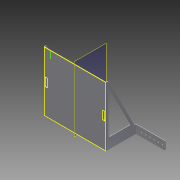
# Autodesk Inventor part: battery mount
Saved by Autodesk Inventor 2014 SP1 (Build 180222100, 222)
## iProperties
Created: 2014-01-05
Part Number: battery mount
Material: Aluminum 6061
Document SubType Name: Sheet Metal
Designer: Arpan
Density: 2.71 g/cm^3
Flat Pattern Width: 54.6969 cm
Flat Pattern Length: 18.034 cm
Flat Pattern Area: 986.403 cm^2
Sheet Metal Rule: Default
Sheet Metal Width: 21.534 in
Sheet Metal Length: 7.100 in
Sheet Metal Area: 152.893 in^2
Appearance: Aluminum - Flat
Mass: 205.427 g
Surface Area: 991.477 cm^2
Volume: 75.8033 cm^3
Author: Arpan
Autodesk Inventor part; units mm, degrees
ref_plane "YZ Plane" through (0, 0, 0) normal (1, 0, 0) x (0, 1, 0)
ref_plane "XZ Plane" through (0, 0, 0) normal (0, 1, 0) x (-1, 0, 0)
ref_plane "XY Plane" through (0, 0, 0) normal (0, 0, 1) x (1, 0, 0)
sketch "Sketch1" plane through (0, 0, 0) normal (0, 0, 1) x (1, 0, 0)
  line L0 (0, 0) -> (-186.69, 0)
  line L1 (-186.69, 0) -> (-186.69, 180.34)
  line L2 (-186.69, 180.34) -> (0, 180.34)
  line L3 (0, 180.34) -> (0, 0)
  line L4 (-186.69, 90.17) -> (-183.515, 90.17)
  line L5 (-183.515, 90.17) -> (-183.515, 102.87)
  line L6 (-183.515, 102.87) -> (-177.165, 102.87)
  line L7 (-177.165, 102.87) -> (-177.165, 77.47)
  line L8 (-177.165, 77.47) -> (-183.515, 77.47)
  line L9 (-183.515, 77.47) -> (-183.515, 90.17)
  line L10 (0, 90.17) -> (-3.175, 90.17)
  line L11 (-3.175, 90.17) -> (-3.175, 102.87)
  line L12 (-3.175, 102.87) -> (-9.525, 102.87)
  line L13 (-9.525, 102.87) -> (-9.525, 77.47)
  line L14 (-9.525, 77.47) -> (-3.175, 77.47)
  line L15 (-3.175, 77.47) -> (-3.175, 90.17)
  dimension "d0" = 180.34
  dimension "d1" = 186.69
  dimension "d2" = 3.175
  dimension "d3" = 12.7
  dimension "d4" = 6.35
  dimension "d5" = 25.4
  dimension "d6" = 3.175
  dimension "d7" = 6.35
  dimension "d8" = 25.4
  measures "d0" distance of L2.end L0.start
  measures "d1" distance of L0.start L0.end
  measures "d2" distance of L4.start L4.end
  measures "d3" distance of L4.end L5.end
  measures "d4" distance of L5.end L6.end
  measures "d5" distance of L6.end L7.end
  measures "d6" distance of L10.start L10.end
  measures "d7" distance of L11.end L12.end
  measures "d8" distance of L12.end L13.end
extrude "Plate1" add sketch "Sketch1" along normal blind 1.5875
sketch "Sketch2" plane through (0.127, 0, -0.127) normal (1, 0, 0) x (0, 1, 0)
  line L0 (180.34, 0) -> (0, 0)
  line L1 (0, 0) -> (0, -88.773)
  line L2 (0, -88.773) -> (180.34, -88.773)
  line L3 (180.34, -88.773) -> (180.34, 0)
  constraints: 6 end point, 1 horizontal, 1 perpendicular, 1 vertical
edge flange "Flange1" height 88.9 angle 90 thickness 1.5875 bend radius 0.127 thickness toward (1, 0, 0) relief straight relief width 1.5875 relief depth 0.7937 corner gap 1.5875 corner form 0 edges at (0, 45.085, 0) (0, 135.255, 0) wall of the first edge with corners at (0.127, 180.34, -0.127) (0.127, 0, -0.127) (0.127, 0, -88.9) (0.127, 180.34, -88.9)
bend "Bend1"
corner "Corner1"
sketch "Sketch3" plane through (-186.817, 180.34, -0.127) normal (-1, 0, 0) x (0, -1, 0)
  line L0 (180.34, 0) -> (0, 0)
  line L1 (0, 0) -> (0, -88.773)
  line L2 (0, -88.773) -> (180.34, -88.773)
  line L3 (180.34, -88.773) -> (180.34, 0)
  constraints: 6 end point, 1 horizontal, 1 perpendicular, 1 vertical
edge flange "Flange2" height 88.9 angle 90 thickness 1.5875 bend radius 0.127 thickness toward (-1, 0, 0) relief straight relief width 1.5875 relief depth 0.7937 edges at (-186.69, 90.17, 0) wall of the first edge with corners at (-186.817, 0, -0.127) (-186.817, 180.34, -0.127) (-186.817, 180.34, -88.9) (-186.817, 0, -88.9)
bend "Bend2"
corner "Corner2"
sketch "Sketch4" plane through (1.8415, 180.34, -89.027) normal (0, 0, -1) x (-1, 0, 0)
  line L0 (0, -180.34) -> (0, 0)
  line L1 (0, 0) -> (-88.773, 0)
  line L2 (-88.773, 0) -> (-88.773, -180.34)
  line L3 (-88.773, -180.34) -> (0, -180.34)
  constraints: 6 end point, 1 horizontal, 1 perpendicular, 1 vertical
edge flange "Flange3" height 88.9 angle 90 thickness 1.5875 bend radius 0.127 thickness toward (0, 0, -1) relief straight relief width 1.5875 relief depth 0.7937 corner gap 1.5875 corner form 0 edges at (1.7145, 90.17, -88.9) (-188.4045, 90.17, -88.9) wall of the first edge with corners at (1.8415, 0, -89.027) (1.8415, 180.34, -89.027) (90.6145, 180.34, -89.027) (90.6145, 0, -89.027)
bend "Bend3"
corner "Corner3"
sketch "Sketch5" plane through (-277.3045, 0, -90.6145) normal (0, 0, -1) x (-1, 0, 0)
  line L0 (0, 180.34) -> (0, 0) projected
  line L1 (-88.773, 180.34) -> (0, 180.34) projected
  line L2 (0, 180.34) -> (-90.4875, 180.34)
  line L3 (-90.4875, 180.34) -> (0, 180.34)
  line L4 (0, 180.34) -> (0, 25.4)
  line L5 (0, 25.4) -> (-90.4875, 25.4)
  line L6 (-90.4875, 25.4) -> (-90.4875, 180.34)
  point P0 (-277.3045, 0)
  dimension "d40" = 90.4875
  dimension "d41" = 154.94
  constraints: 10 end point, 2 parallel, 2 point on line, 1 horizontal, 1 perpendicular
  measures "d40" distance of L0.start L2.end
  measures "d41" distance of L3.end L4.end
extrude "Cut1" cut sketch "Sketch5" against normal blind 6.35
sketch "Sketch6" plane through (90.6145, 0, -90.6145) normal (0, 0, -1) x (-1, 0, 0)
  line L0 (0, 180.34) -> (90.5002, 180.34)
  line L1 (90.5002, 180.34) -> (90.5002, 25.4)
  line L2 (90.5002, 25.4) -> (0, 25.4)
  line L3 (0, 25.4) -> (0, 180.34)
  point P0 (90.6145, 0)
  dimension "d44" = 90.5002
  dimension "d45" = 154.94
  constraints: 8 end point, 2 parallel, 1 horizontal, 1 perpendicular
  measures "d44" distance of L1.end L2.end
  measures "d45" distance of L2.end L0.start
extrude "Cut2" cut sketch "Sketch6" against normal blind 6.35
sketch "Sketch7" plane through (-188.4045, 0, -0.127) normal (-1, 0, 0) x (0, 0, 1)
  line L0 (-84.1375, 180.34) -> (0, 180.34) projected
  line L1 (-84.1375, 180.34) -> (-84.1375, 25.4) projected
  line L2 (0, 180.34) -> (-6.35, 180.34)
  line L3 (-6.35, 180.34) -> (-84.1375, 25.4)
  point P0 (0.127, 0)
  dimension "d48" = 6.35
  constraints: 4 end point, 1 point on line
  measures "d48" distance of L0.end L2.end
extrude "Cut3" cut sketch "Sketch7" against normal blind 1.5875
sketch "Sketch8" plane through (1.7145, 0, -0.127) normal (1, 0, 0) x (0, 0, -1)
  line L0 (84.1375, 25.4) -> (84.1375, 180.34) projected
  line L1 (0, 180.34) -> (84.1375, 180.34) projected
  line L2 (0, 180.34) -> (6.35, 180.34)
  line L3 (6.35, 180.34) -> (84.1375, 25.4)
  point P0 (-0.127, 0)
  dimension "d51" = 6.35
  constraints: 4 end point, 1 point on line
  measures "d51" distance of L1.start L2.end
extrude "Cut4" cut sketch "Sketch8" against normal blind 1.5875
fillet "Corner Round1" radius 3.175 4 edges at (0.9207, 180.34, -6.477) (-187.6108, 180.34, -6.477) (-187.6108, 25.4, -84.2645) (0.9207, 25.4, -84.2645)
fillet "Corner Round2" radius 3.175 4 edges at (90.6145, 25.4, -89.8207) (90.6145, 0, -89.8207) (-277.3045, 25.4, -89.8208) (-277.3045, 0, -89.8208)
sketch "Sketch9" plane through (-188.4045, 0, -0.127) normal (-1, 0, 0) x (0, 0, 1)
  line L0 (-7.2288, 178.5896) -> (-83.2587, 27.1504) projected
  line L1 (0, 0) -> (0, 180.34) projected
  line L2 (0, 25.4) -> (0, 31.75)
  line L3 (-73.8441, 31.75) -> (-6.35, 166.1873)
  line L4 (-6.35, 166.1873) -> (-6.35, 31.75)
  line L5 (-6.35, 31.75) -> (-73.8441, 31.75)
  point P0 (0.127, 0)
  dimension "d56" = 6.35
  dimension "d57" = 6.35
  dimension "d58" = 6.35
  constraints: 8 end point, 2 point on line, 1 perpendicular
  measures "d56" distance of L2.start L2.end
  measures "d57" distance between parallel lines of L0 L3
  measures "d58" distance between parallel lines of L1 L4
extrude "Cut5" cut sketch "Sketch9" against normal blind 1.5875
sketch "Sketch10" plane through (1.7145, 0, -0.127) normal (1, 0, 0) x (0, 0, -1)
  line L0 (73.8441, 31.75) -> (6.35, 31.75) projected
  line L1 (6.35, 31.75) -> (6.35, 166.1873) projected
  line L2 (6.35, 166.1873) -> (73.8441, 31.75) projected
  point P0 (-0.127, 0)
extrude "Cut6" cut sketch "Sketch10" against normal blind 1.5875
fillet "Corner Round3" radius 3.175 6 edges at (0.9208, 31.75, -6.477) (0.9208, 31.75, -73.9711) (0.9207, 166.1873, -6.477) (-187.6108, 166.1873, -6.477) (-187.6108, 31.75, -6.477) (-187.6108, 31.75, -73.9711)
sketch "Sketch12" plane through (0, 0, 1.5875) normal (0, 0, 1) x (1, 0, 0)
  line L0 (-183.515, 77.47) -> (-183.515, 102.87) projected
  line L1 (-183.515, 102.87) -> (-177.165, 102.87) projected
  line L2 (-177.165, 102.87) -> (-177.165, 77.47) projected
  line L3 (-177.165, 77.47) -> (-183.515, 77.47) projected
  line L4 (-3.175, 102.87) -> (-3.175, 77.47) projected
  line L5 (-3.175, 77.47) -> (-9.525, 77.47) projected
  line L6 (-9.525, 77.47) -> (-9.525, 102.87) projected
  line L7 (-9.525, 102.87) -> (-3.175, 102.87) projected
  line L8 (0, 0) -> (-186.69, 0) projected
  line L9 (0, 180.34) -> (0, 0) projected
  line L10 (-186.69, 180.34) -> (0, 180.34) projected
  line L11 (-186.69, 0) -> (-186.69, 180.34) projected
  line L12 (-167.3882, 159.3651) -> (-167.3882, 180.34)
  constraints: 2 end point, 1 point on line
sketch "Sketch14" plane through (-188.5315, 0, -89.027) normal (0, 0, 1) x (1, 0, 0)
  line L0 (-88.773, 22.225) -> (-88.773, 3.175) projected
  line L1 (-88.773, 12.7) -> (-79.248, 12.7)
  circle A0 centre (-79.248, 12.7) radius 2.4257
  point P0 (188.5315, 0)
  dimension "d66" = 9.525
  dimension "d67" = 4.8514
  constraints: 2 end point, 1 centre point, 1 coincident, 1 midpoint, 1 perpendicular
  measures "d66" distance of L1.start L1.end
  measures "d67" diameter of A0
extrude "Cut8" cut sketch "Sketch14" against normal blind 1.5875
pattern_linear "Rectangular Pattern2" count 6 spacing 12.7 along (1, 0, 0) of "Cut8"
ref_plane "Work Plane1" through (-92.837, 0, -0.127) normal (-1, 0, 0) x (0, 0, 1)
mirror "Mirror1" about plane through (-92.837, 0, -0.127) normal (-1, 0, 0) of "Cut8", "Rectangular Pattern2"
equation "\"d49\" = Thickness"
equation "\"d52\" = Thickness"
equation "\"d59\" = Thickness"
equation "\"d61\" = Thickness"
equation "\"d68\" = Thickness"
equation "\"d10\" = BendReliefWidth"
equation "\"d11\" = BendReliefDepth"
equation "\"d12\" = MinimumRemnant"
equation "\"d13\" = BendRadius"
equation "\"d17\" = CornerReliefSize"
equation "\"d18\" = GapSize"
equation "\"d19\" = JacobiRadiusSize"
equation "\"d20\" = BendReliefWidth"
equation "\"d21\" = BendReliefDepth"
equation "\"d22\" = MinimumRemnant"
equation "\"d23\" = BendRadius"
equation "\"d27\" = CornerReliefSize"
equation "\"d28\" = GapSize"
equation "\"d29\" = JacobiRadiusSize"
equation "\"d30\" = BendReliefWidth"
equation "\"d31\" = BendReliefDepth"
equation "\"d32\" = MinimumRemnant"
equation "\"d33\" = BendRadius"
equation "\"d37\" = CornerReliefSize"
equation "\"d38\" = GapSize"
equation "\"d39\" = JacobiRadiusSize"
equation "\"BendRadius\" = Thickness"
equation "\"BendReliefWidth\" = Thickness"
equation "\"BendReliefDepth\" = 0.5 * Thickness"
equation "\"CornerReliefSize\" = 4 * Thickness"
equation "\"MinimumRemnant\" = 2 * Thickness"
equation "\"TransitionRadius\" = BendRadius"
equation "\"JacobiRadiusSize\" = BendRadius"
equation "\"GapSize\" = Thickness"
equation "\"d9\" = BendRadius"
equation "\"Thickness\" = 1.5875"
body "Solid1"
